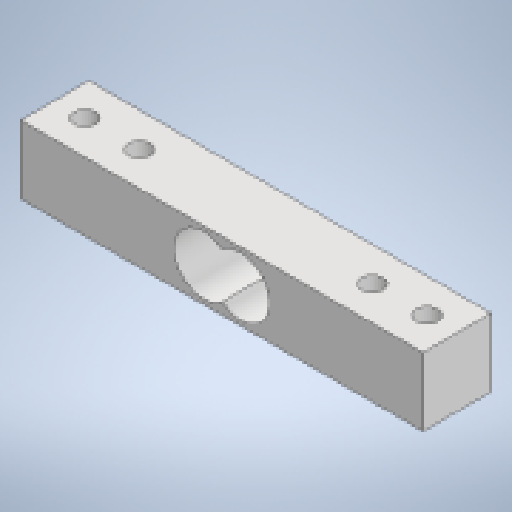
# Autodesk Inventor part: Celda_Carga
Saved by Autodesk Inventor 2024 (Build 280153000, 153)
## iProperties
Created: 2024-07-16
Part Number: Celda_Carga
Material: Genérico
Document SubType Name: Modeling
Designer: sergi
Density: 1 g/cm^3
Appearance: Valor por defecto
Author: sergi
Autodesk Inventor part; units mm, degrees
ref_plane "YZ Plane" through (0, 0, 0) normal (1, 0, 0) x (0, 1, 0)
ref_plane "XZ Plane" through (0, 0, 0) normal (0, 1, 0) x (-1, 0, 0)
ref_plane "XY Plane" through (0, 0, 0) normal (0, 0, 1) x (1, 0, 0)
sketch "Boceto1" plane through (0, 0, 0) normal (0, 0, 1) x (1, 0, 0)
  line L0 (0, 0) -> (75, 0)
  line L1 (75, 0) -> (75, 12.7)
  line L2 (75, 12.7) -> (0, 12.7)
  line L3 (0, 12.7) -> (0, 0)
  dimension "d0" = 75
  dimension "d1" = 12.7
  constraints: 8 end point, 2 parallel, 1 horizontal, 1 perpendicular
  measures "d0" distance of L2.end L1.end
  measures "d1" distance of L1.end L0.end
extrude "Extrusión1" add sketch "Boceto1" along normal blind 12.7
sketch "Boceto2" plane through (0, 0, 0) normal (0, 0, -1) x (-1, 0, 0)
  line L0 (0, 12.7) -> (0, 0) projected
  line L1 (0, 6.35) -> (-28.6, 6.35)
  line L2 (-28.6, 6.35) -> (-34.05, 6.35)
  line L3 (-28.6, 6.35) -> (-23.15, 6.35) construction
  circle A0 centre (-34.05, 6.35) radius 5.45
  line L4 (-75, 6.35) -> (-46.4, 6.35)
  line L5 (-46.4, 6.35) -> (-40.95, 6.35)
  line L6 (-46.4, 6.35) -> (-51.85, 6.35) construction
  circle A1 centre (-40.95, 6.35) radius 5.45
  point P0 (-37.5, 2.131)
  point P1 (-37.5, 10.569)
  dimension "d4" = 28.6
  dimension "d5" = 5.45
  dimension "d6" = 180
  dimension "d7" = 28.6
  dimension "d8" = 5.45
  dimension "d9" = 180
  constraints: 12 end point, 3 horizontal, 2 coincident, 2 collinear, 1 midpoint, 6 other
  measures "d4" distance of L1.start L1.end
  measures "d5" distance of L1.end L2.end
  measures "d6" angle of L2 L3
  measures "d7" distance of L4.start L4.end
  measures "d8" distance of L4.end L5.end
  measures "d9" angle of L5 L6
extrude "Extrusión2" cut sketch "Boceto2" against normal blind 12.7
sketch "Boceto3" plane through (0, 0, 0) normal (0, -1, 0) x (1, 0, 0)
  line L0 (75, 0) -> (75, 12.7) projected
  line L1 (75, 6.35) -> (71.1, 6.35)
  line L2 (71.1, 6.35) -> (69.375, 6.35)
  circle A0 centre (69.375, 6.35) radius 1.725
  line L3 (67.65, 6.35) -> (60.9, 6.35)
  line L4 (60.9, 6.35) -> (59.175, 6.35)
  circle A1 centre (59.175, 6.35) radius 1.725
  circle A2 centre (69.375, 6.35) radius 2
  circle A3 centre (59.175, 6.35) radius 2
  line L5 (75, 0) -> (0, 0) projected
  line L6 (37.5, 0) -> (37.5, 12.7)
  line L7 (0, 12.7) -> (75, 12.7) projected
  line L8 (0, 6.4) -> (3.9, 6.4)
  line L9 (3.9, 6.4) -> (5.625, 6.4)
  circle A4 centre (5.625, 6.4) radius 1.725
  line L10 (7.35, 6.4) -> (14.1, 6.4)
  line L11 (14.1, 6.4) -> (15.825, 6.4)
  circle A5 centre (15.825, 6.4) radius 1.725
  circle A6 centre (5.625, 6.4) radius 2
  circle A7 centre (15.825, 6.4) radius 2
  line L12 (0, 0) -> (75, 0) projected
  dimension "d12" = 3.9
  dimension "d13" = 1.725
  dimension "d14" = 6.75
  dimension "d15" = 1.725
  dimension "d16" = 4
  dimension "d17" = 4
  dimension "d18" = 3.9
  dimension "d19" = 1.725
  dimension "d20" = 6.75
  dimension "d21" = 1.725
  dimension "d22" = 4
  dimension "d23" = 4
  dimension "d31" = 6.4
  dimension "d32" = 6.4
  constraints: 18 end point, 8 coincident, 6 centre point, 4 horizontal, 4 point on circle, 3 midpoint, 2 horizontal alignment, 4 other
  measures "d12" distance of L1.start L1.end
  measures "d13" distance of L1.end L2.end
  measures "d14" distance of L3.start L3.end
  measures "d15" distance of L3.end L4.end
  measures "d16" diameter of A2
  measures "d17" diameter of A3
  measures "d18" distance of L8.start L8.end
  measures "d19" distance of L8.end L9.end
  measures "d20" distance of L10.start L10.end
  measures "d21" distance of L10.end L11.end
  measures "d22" diameter of A6
  measures "d23" diameter of A7
  measures "d31" distance between parallel lines of L12 L10
  measures "d32" distance between parallel lines of L12 L9
hole "Agujero1" at (59.175, 0, 6.35) at (69.375, 0, 6.35) at (15.825, 0, 6.4) at (5.625, 0, 6.4) direction (0, 1, 0) diameter 4 depth 12.7
